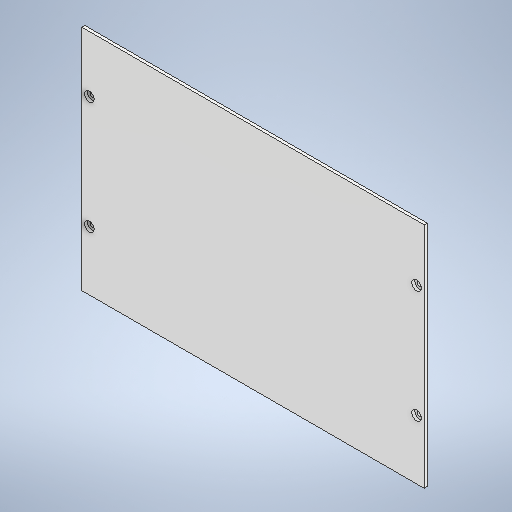
# Autodesk Inventor part: Lid
Saved by Autodesk Inventor 2025 (Build 290162000, 162)
## iProperties
Created: 2025-05-20
Part Number: Lid
Material: Generic
Document SubType Name: Modeling
Designer: ethan
Density: 1 g/cm^3
Appearance: PTFE(1)
Author: ethan
Autodesk Inventor part; units mm, degrees
ref_plane "YZ Plane" through (0, 0, 0) normal (1, 0, 0) x (0, 1, 0)
ref_plane "XZ Plane" through (0, 0, 0) normal (0, 1, 0) x (-1, 0, 0)
ref_plane "XY Plane" through (0, 0, 0) normal (0, 0, 1) x (1, 0, 0)
sketch "Sketch1" plane through (0, 0, 0) normal (0, 0, 1) x (1, 0, 0)
  circle A0 centre (0, -37.6) radius 2.25 construction
  circle A1 centre (0, 37.6) radius 2.25 construction
  line L0 (-3, 73.2) -> (-3, -73.2) construction
  line L1 (3, -73.2) -> (-3, -73.2) construction
  line L2 (3, 73.2) -> (3, -73.2) construction
  line L3 (-3, 73.2) -> (3, 73.2) construction
  line L4 (3, 73.2) -> (-3, 73.2) construction
  line L5 (-3, 73.2) -> (-3, 75.2) construction
  line L6 (-3, 75.2) -> (3, 75.2) construction
  line L7 (3, 75.2) -> (3, 73.2) construction
  line L8 (3, -73.2) -> (-221.6, -73.2) construction
  line L9 (-221.6, -73.2) -> (-221.6, 73.2) construction
  line L10 (-221.6, 73.2) -> (3, 73.2) construction
  line L11 (3, 73.2) -> (3, -73.2) construction
  line L12 (3, 75.2) -> (-221.6, 75.2)
  line L13 (-221.6, 75.2) -> (-221.6, -73.2)
  line L14 (-221.6, -73.2) -> (3, -73.2)
  line L15 (3, -73.2) -> (3, 75.2)
  point P0 (0, 0)
  dimension "d0" = 2
  dimension "d1" = 224.6
  constraints: 24 end point, 6 parallel, 3 horizontal, 3 perpendicular
  measures "d0" distance of L4.end L5.end
  measures "d1" distance of L9.end L10.end
extrude "Extrusion1" add sketch "Sketch1" along normal blind 2
sketch "Sketch2" plane through (0, 0, 2) normal (0, 0, 1) x (1, 0, 0)
  line L0 (-221.6, 75.2) -> (-221.6, -73.2) construction
  line L1 (-221.6, -73.2) -> (3, -73.2) construction
  line L2 (3, -73.2) -> (3, 75.2) construction
  line L3 (3, 75.2) -> (-221.6, 75.2) construction
  line L4 (5, 77.2) -> (5, -75.2)
  line L5 (5, -75.2) -> (-223.6, -75.2)
  line L6 (-223.6, -75.2) -> (-223.6, 77.2)
  line L7 (-223.6, 77.2) -> (5, 77.2)
  point P0 (0, 0)
  dimension "d4" = 2
  constraints: 8 end point, 3 other
  measures "d4" distance between parallel lines of L2 L4
extrude "Extrusion2" add sketch "Sketch2" along normal blind 2
sketch "Sketch4" plane through (0, 0, 4) normal (0, 0, 1) x (1, 0, 0)
  circle A0 centre (0, -35.6) radius 2.25 construction
  circle A1 centre (0, 39.6) radius 2.25 construction
  line L0 (-3, 75.2) -> (-3, -71.2) construction
  line L1 (3, -71.2) -> (-3, -71.2) construction
  line L2 (3, 75.2) -> (3, -71.2) construction
  line L3 (-3, 75.2) -> (3, 75.2) construction
  circle A2 centre (-218.6, 39.6) radius 2.25 construction
  circle A3 centre (-218.6, -35.6) radius 2.25 construction
  line L4 (-215.6, -71.2) -> (-215.6, 75.2) construction
  line L5 (-221.6, 75.2) -> (-215.6, 75.2) construction
  line L6 (-221.6, -71.2) -> (-221.6, 75.2) construction
  line L7 (-215.6, -71.2) -> (-221.6, -71.2) construction
  circle A4 centre (0, -35.6) radius 3.25
  circle A5 centre (0, 39.6) radius 3.25
  circle A6 centre (-218.6, -35.6) radius 3.25
  circle A7 centre (-218.6, 39.6) radius 3.25
  point P0 (0, 0)
  dimension "d7" = 1
  dimension "d8" = 1
  dimension "d9" = 1
  dimension "d10" = 1
  constraints: 4 centre point
  measures "d7" radial gap between concentric circles of A0 A4
  measures "d8" radial gap between concentric circles of A1 A5
  measures "d9" radial gap between concentric circles of A3 A6
  measures "d10" radial gap between concentric circles of A2 A7
extrude "Extrusion3" cut sketch "Sketch4" against normal blind 2
sketch "Sketch5" plane through (0, 0, 2) normal (0, 0, 1) x (1, 0, 0)
  line L0 (3, -36.85) -> (3, -34.35) projected
  arc A0 (3, -34.35) -> (3, -36.85) centre (0, -35.6) ccw projected
  line L1 (3, 38.35) -> (3, 40.85) projected
  arc A1 (3, 40.85) -> (3, 38.35) centre (0, 39.6) ccw projected
  line L2 (-221.6, -34.35) -> (-221.6, -36.85) projected
  arc A2 (-221.6, -36.85) -> (-221.6, -34.35) centre (-218.6, -35.6) ccw projected
  line L3 (-221.6, 40.85) -> (-221.6, 38.35) projected
  arc A3 (-221.6, 38.35) -> (-221.6, 40.85) centre (-218.6, 39.6) ccw projected
  circle A4 centre (-218.6, 39.6) radius 1.6
  circle A5 centre (-218.6, -35.6) radius 1.6
  circle A6 centre (0, -35.6) radius 1.6
  circle A7 centre (0, 39.6) radius 1.6
  point P0 (0, 0)
  dimension "d13" = 3.2
  dimension "d14" = 3.2
  dimension "d15" = 3.2
  dimension "d16" = 3.2
  constraints: 4 centre point, 4 coincident
  measures "d13" diameter of A4
  measures "d14" diameter of A5
  measures "d15" diameter of A6
  measures "d16" diameter of A7
extrude "Extrusion4" cut sketch "Sketch5" against normal blind 2 contours A4 | A5 | A6 | A7
body "Solid1"
